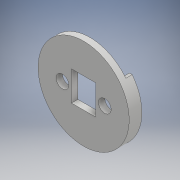
# Autodesk Inventor part: EndCapProper
Saved by Autodesk Inventor 2018 (Build 220112000, 112)
## iProperties
Created: 2018-05-20
Part Number: EndCapProper
Material: Generic
Document SubType Name: Modeling
Designer: a
Density: 1 g/cm^3
Appearance: Default
Author: a
## iProperties of the stored document EndCap_3DPrint.ipt
Created: 2018-05-20
Part Number: EndCap_3DPrint
Material: Generic
Document SubType Name: Modeling
Designer: a
Density: 1 g/cm^3
Appearance: Default
Author: a
Autodesk Inventor part; units mm, degrees
ref_plane "YZ Plane" through (0, 0, 0) normal (1, 0, 0) x (0, 1, 0)
ref_plane "XZ Plane" through (0, 0, 0) normal (0, 1, 0) x (-1, 0, 0)
ref_plane "XY Plane" through (0, 0, 0) normal (0, 0, 1) x (1, 0, 0)
sketch "Sketch1" plane through (0, 0, 0) normal (0, 1, 0) x (-1, 0, 0)
  circle A0 centre (0, 0) radius 21.5
  dimension "d1" = 43
  constraints: 1 centre point
  measures "d1" diameter of A0
extrude "Extrusion1" add sketch "Sketch1" along normal blind 3
sketch "Sketch2" plane through (0, 3, 0) normal (0, 1, 0) x (1, 0, 0)
  arc A0 (15.6228, -13.2732) -> (-15.6228, -13.2732) centre (0, 0) ccw
  arc A1 (16.9137, -13.2732) -> (-16.9137, -13.2732) centre (0, 0) ccw
  circle A2 centre (0, 0) radius 21.5 projected
  line L0 (-16.9137, -13.2732) -> (-15.6228, -13.2732)
  line L1 (15.6228, -13.2732) -> (16.9137, -13.2732)
  dimension "d4" = 41
  constraints: 6 point on circle, 4 end point, 2 centre point, 2 coincident, 2 horizontal
  measures "d4" diameter of A0
extrude "Extrusion2" add sketch "Sketch2" along normal blind 3 contours A0 L0 A1 L1
sketch "Sketch3" plane through (0, 3, 0) normal (0, 1, 0) x (1, 0, 0)
  circle A0 centre (-10, 0) radius 3
  circle A1 centre (10, 0) radius 3
  point P0 (0, 0)
  dimension "d7" = 6
  dimension "d8" = 6
  constraints: 2 centre point
  measures "d7" diameter of A0
  measures "d8" diameter of A1
extrude "Extrusion3" cut sketch "Sketch3" against normal blind 10 contours A0
sketch "Sketch4" plane through (0, 3, 0) normal (0, 1, 0) x (1, 0, 0)
  circle A0 centre (10, 0) radius 3
  point P0 (0, 0)
  dimension "d11" = 6
  constraints: 1 centre point
  measures "d11" diameter of A0
extrude "Extrusion4" cut sketch "Sketch4" against normal blind 10
sketch "Sketch5" plane through (0, 3, 0) normal (0, 1, 0) x (1, 0, 0)
  line L0 (0, 6) -> (5, 6)
  line L1 (5, 6) -> (5, -6)
  line L2 (5, -6) -> (-5, -6)
  line L3 (-5, -6) -> (-5, 6)
  line L4 (-5, 6) -> (0, 6)
  point P0 (0, 0)
  constraints: 10 end point, 3 perpendicular, 1 collinear, 1 point on line
extrude "Extrusion5" cut sketch "Sketch5" against normal blind 10
sketch "Sketch6" plane through (0, 3, 0) normal (0, 1, 0) x (1, 0, 0)
  line L0 (5, 6) -> (5.7071, 6.7071)
  line L1 (5, 6) -> (6, 6) construction
  line L2 (5.7071, 6.7071) -> (5.7071, -7.2929)
  line L3 (5.7071, -7.2929) -> (-5.7269, -7.2929)
  line L4 (-5.7269, -7.2929) -> (-5.7269, 6.7071)
  line L5 (-5.7269, 6.7071) -> (5.7071, 6.7071)
  point P0 (0, 0)
  dimension "d21" = 1
  dimension "d22" = 45
  dimension "d23" = 14
  dimension "d24" = 45
  constraints: 12 end point, 3 perpendicular, 1 equal length, 1 horizontal, 1 vertical
  measures "d21" distance of L0.start L0.end
  measures "d22" angle of L1 L0
  measures "d23" distance of L0.end L2.end
  measures "d24" angle of L0 L2
extrude "Extrusion6" cut sketch "Sketch6" against normal blind 10
body "Solid1"
